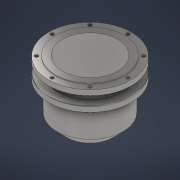
# Autodesk Inventor part: 003
Saved by Autodesk Inventor 2022 (Build 260153000, 153)
## iProperties
Created: 2021-11-04
Part Number: 003
Material: Stainless Steel, 440C
Document SubType Name: Modeling
Designer: vinicius.miguel
Density: 7.75 g/cm^3
Appearance: Semi-Polished
Mass: 2079.97 g
Surface Area: 727.794 cm^2
Volume: 268.384 cm^3
Author: vinicius.miguel
Autodesk Inventor part; units mm, degrees
ref_plane "YZ Plane" through (0, 0, 0) normal (1, 0, 0) x (0, 1, 0)
ref_plane "XZ Plane" through (0, 0, 0) normal (0, 1, 0) x (-1, 0, 0)
ref_plane "XY Plane" through (0, 0, 0) normal (0, 0, 1) x (1, 0, 0)
sketch "Sketch1" plane through (0, 0, 0) normal (0, 0, 1) x (1, 0, 0)
  line L0 (23.75, 0.7) -> (25, 0.7)
  line L1 (25, 0.7) -> (25, 0)
  line L2 (25, 0) -> (32.5, 0)
  line L3 (32.5, 0) -> (48, 15.5)
  line L4 (48, 15.5) -> (48, 57.5)
  line L5 (48, 57.5) -> (60, 57.5)
  line L6 (60, 57.5) -> (60, 87.5)
  line L7 (60, 87.5) -> (40, 87.5)
  line L8 (40, 87.5) -> (40, 20)
  line L9 (40, 20) -> (35.81, 20)
  line L10 (35.81, 20) -> (23.75, 0.7)
  line L11 (0, 0) -> (0, 69.5074) construction
  line L12 (50, 87.5) -> (50, 86.5)
  line L13 (50, 86.5) -> (60, 86.5)
  line L14 (48, 57.5) -> (48, 59.8)
  line L15 (48, 59.8) -> (52, 59.8)
  line L16 (52, 59.8) -> (52, 57.5)
  line L17 (60, 78.5) -> (48, 78.5)
  line L18 (48, 78.5) -> (48, 65.8)
  line L19 (48, 65.8) -> (60, 65.8)
  dimension "d0" = 135
  dimension "d2" = 80
  dimension "d3" = 50
  dimension "d4" = 47.5
  dimension "d5" = 65
  dimension "d6" = 20
  dimension "d9" = 30
  dimension "d10" = 120
  dimension "d11" = 0.7
  dimension "d13" = 122
  dimension "d26" = 1
  dimension "d27" = 100
  dimension "d28" = 96
  dimension "d29" = 4
  dimension "d30" = 2.3
  dimension "d31" = 87.5
  dimension "d32" = 6
  dimension "d33" = 8
  constraints: 40 end point, 12 perpendicular, 4 point on line, 3 vertical, 2 horizontal, 1 horizontal alignment, 1 midpoint, 1 parallel, 1 vertical alignment
  measures "d0" angle of L2 L3
  measures "d2" diameter of L8 L11
  measures "d3" diameter of L1 L11
  measures "d4" diameter of L0.start L11
  measures "d5" diameter of L2.end L11
  measures "d6" distance from line of L11.start L9
  measures "d9" distance of L5.end L6.end
  measures "d10" diameter of L6 L11
  measures "d11" distance of L0.end L1.end
  measures "d13" angle of L10 L0
  measures "d26" distance of L12.start L12.end
  measures "d27" diameter of L12 L11
  measures "d28" diameter of L4 L11
  measures "d29" distance of L14.end L15.end
  measures "d30" distance of L4.end L14.end
  measures "d31" distance from line of L7 L11.start
  measures "d32" distance between parallel lines of L19 L15
  measures "d33" distance between parallel lines of L13 L17
revolve "Revolution1" add sketch "Sketch1" angle 360 about axis through (0, 0, 0) along (0, 1, 0) contours L10 L9 L8 L7 L12 L13 L6 L17 L18 L19 L5 L16 L15 L14 L4 L3 L2 L1 L0
sketch "Sketch2" plane through (0, 86.5, 0) normal (0, 1, 0) x (1, 0, 0)
  circle A0 centre (55, 0) radius 4
  point P0 (0, 0)
  dimension "d14" = 55
  dimension "d25" = 8
  constraints: 1 centre point, 1 coincident, 1 horizontal alignment
  measures "d14" distance of point (55, 0) point (0, 0)
  measures "d25" diameter of A0
hole "Hole1" at (55, 86.5, 0) direction (0, -1, 0) diameter 4.917 depth 8 tip angle 118 thread size "M6x1" class "6H" standard "ISO Metric profile"
pattern_circular "Circular Pattern1" count 8 over 360 about axis through (0, 37.65, 0) along (0, -1, 0) of "Hole1"
chamfer "Chamfer1" distance 0.5 angle 45 3 edges at (-60, 65.8, 0) (-60, 57.5, 0) (-60, 78.5, 0)
sketch "Sketch3" plane through (0, 0, 0) normal (0, -1, 0) x (1, 0, 0)
  point P0 (0, 0)
  point P1 (29.5, 0)
  dimension "d37" = 29.5
  constraints: 1 horizontal alignment
  measures "d37" distance of point (29.5, 0) point (0, 0)
hole "Hole2" at (29.5, 0, 0) direction (0, 1, 0) diameter 1.567 depth 5 tip angle 118 thread size "M2x0.4" class "6H" standard "ISO Metric profile"
pattern_circular "Circular Pattern2" count 4 over 360 about axis through (0, 37.65, 0) along (0, -1, 0) of "Hole2"
body "Solid1"
